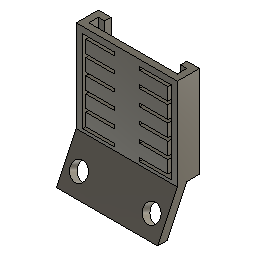
clip (Autodesk Fusion 360 design; units mm, degrees)
Autodesk Fusion 360 part; units mm, degrees
sketch "Skizze1" plane through (0, 0, 0) normal (1, 0, 0) x (0, 1, 0)
  line L0 (5, 36) -> (5, 7)
  line L1 (5, 7) -> (1, 7)
  line L2 (5, 36) -> (-2, 36)
  line L3 (-9.0346, 36) -> (15, -14) construction
  line L4 (-5.2641, -6.0314) -> (1, 7)
  line L5 (-2, 7) -> (-8.2641, -6.0314)
  line L6 (-8.2641, -6.0314) -> (-5.2641, -6.0314)
  line L7 (-2, 7) -> (-2, 36)
  constraint vertical L0
  constraint perpendicular L0 L1
  constraint horizontal L2
extrude "Extrusion2" add sketch "Skizze1" along normal mid plane 32 makes body 1
sketch "Skizze2" plane through (0, 0, 36) normal (0, 0, 1) x (-1, 0, 0)
  line L0 (-16, 2) -> (-16, -5)
  line L1 (-16, -5) -> (16, -5)
  line L2 (16, -5) -> (16, 2)
  line L3 (12, -3) -> (14, -3)
  line L4 (14, -3) -> (14, -1)
  line L5 (14, -1) -> (-14, -1)
  line L6 (-14, -1) -> (-14, -3)
  line L7 (-14, -3) -> (-12, -3)
  line L8 (-12, -3) -> (-12, -5)
  line L9 (12, -3) -> (12, -5)
  line L10 (12, -5) -> (-12, -5)
  line L11 (16, 2) -> (-16, 2)
  line L12 (12, -3) -> (-12, -3)
  constraint parallel L1 L3
  constraint perpendicular L1 L4
  constraint perpendicular L4 L5
  constraint perpendicular L1 L6
  constraint perpendicular L6 L7
  constraint coincident L1 L8.end
  constraint perpendicular L1 L8
  constraint coincident L1 L9.end
  constraint perpendicular L1 L9
  constraint perpendicular L8 L12
extrude "Extrusion3" cut sketch "Skizze2" against normal blind 28 contours L1 L8 L9 L10 L12 | L3 L4 L5 L6 L7 L12 bodies 1
sketch "Skizze3" plane through (0, -2, 0) normal (0, -1, 0) x (1, 0, 0)
  line L0 (-4, 29) -> (-4, 28)
  line L1 (-4, 28) -> (-13, 28)
  line L2 (-13, 28) -> (-13, 24)
  line L3 (-13, 24) -> (-4, 24)
  line L4 (-4, 24) -> (-4, 23)
  line L5 (-4, 23) -> (-13, 23)
  line L6 (-13, 23) -> (-13, 19)
  line L7 (-13, 19) -> (-4, 19)
  line L8 (-4, 19) -> (-4, 18)
  line L9 (-4, 18) -> (-13, 18)
  line L10 (-13, 18) -> (-13, 14)
  line L11 (-13, 14) -> (-4, 14)
  line L12 (-4, 14) -> (-4, 13)
  line L13 (-4, 13) -> (-13, 13)
  line L14 (-13, 13) -> (-13, 9)
  line L15 (-13, 9) -> (-4, 9)
  line L16 (-4, 9) -> (-4, 8)
  line L17 (-4, 8) -> (-14, 8)
  line L18 (-4, 29) -> (-13, 29)
  line L19 (-13, 29) -> (-13, 33)
  line L20 (-13, 33) -> (-4, 33)
  line L21 (-4, 33) -> (-4, 34)
  line L22 (-4, 34) -> (-14, 34)
  line L23 (-14, 34) -> (-14, 8)
  line L24 (4, 9) -> (4, 8)
  line L25 (4, 23) -> (13, 23)
  line L26 (4, 18) -> (13, 18)
  line L27 (4, 8) -> (14, 8)
  line L28 (13, 18) -> (13, 14)
  line L29 (4, 14) -> (4, 13)
  line L30 (14, 34) -> (14, 8)
  line L31 (13, 23) -> (13, 19)
  line L32 (4, 28) -> (13, 28)
  line L33 (4, 33) -> (4, 34)
  line L34 (13, 28) -> (13, 24)
  line L35 (13, 19) -> (4, 19)
  line L36 (13, 29) -> (13, 33)
  line L37 (13, 33) -> (4, 33)
  line L38 (4, 34) -> (14, 34)
  line L39 (4, 24) -> (4, 23)
  line L40 (4, 29) -> (4, 28)
  line L41 (13, 9) -> (4, 9)
  line L42 (4, 19) -> (4, 18)
  line L43 (13, 13) -> (13, 9)
  line L44 (4, 13) -> (13, 13)
  line L45 (13, 14) -> (4, 14)
  line L46 (13, 24) -> (4, 24)
  line L47 (4, 29) -> (13, 29)
  line L48 (-16, 7) -> (16, 7)
  line L49 (16, 7) -> (16, 36)
  line L50 (16, 36) -> (-16, 36)
  line L51 (-16, 36) -> (-16, 7)
  constraint perpendicular L0 L1
  constraint perpendicular L1 L2
  constraint perpendicular L0 L3
  constraint perpendicular L1 L4
  constraint perpendicular L0 L5
  constraint perpendicular L1 L6
  constraint perpendicular L6 L7
  constraint perpendicular L7 L8
  constraint perpendicular L6 L9
  constraint perpendicular L9 L10
  constraint perpendicular L6 L11
  constraint perpendicular L11 L12
  constraint perpendicular L12 L13
  constraint perpendicular L11 L14
  constraint perpendicular L14 L15
  constraint perpendicular L11 L16
  constraint perpendicular L16 L17
  constraint perpendicular L0 L18
  constraint perpendicular L18 L19
  constraint perpendicular L0 L20
  constraint perpendicular L20 L21
  constraint perpendicular L0 L22
  constraint perpendicular L17 L23
extrude "Extrusion4" cut sketch "Skizze3" against normal blind 3 contours L0 L1 L2 L3 L4 L5 L6 L7 L8 L9 L10 L11 L12 L13 L14 L15 L16 L17 L18 L19 L20 L21 L22 L23 | L24 L25 L26 L27 L28 L29 L30 L31 L32 L33 L34 L35 L36 L37 L38 L39 L40 L41 L42 L43 L44 L45 L46 L47 bodies 1
sketch "Skizze4" plane through (-13, 0, 0) normal (-1, 0, 0) x (0, -1, 0)
  spline S0 degree 5 poles (-0.6, 30) (-0.5838, 30.0067) (-0.5435, 30.0228) (-0.4594, 30.0556) (-0.3079, 30.1256) (-0.0957, 30.3027) (0.0811, 30.5925) (0.1688, 30.9921) (0.1107, 31.3665) (-0.0858, 31.6037) (-0.3409, 31.7375) (-0.5133, 31.8156) (-0.5842, 31.895) (-0.6, 31.9626) (-0.6, 32) knots 0 0 0 0 0 0 0.1 0.2 0.3 0.4 0.5 0.6 0.7 0.8 0.9 1 1 1 1 1 1
  line L0 (-0.6964, 29.9603) -> (-0.5036, 30.0397)
  line L1 (-0.6, 31.7862) -> (-0.6, 32.2138)
  line L2 (0, 33.0963) -> (-1, 33.0963)
  line L3 (-1, 33.0963) -> (-1, 28.9104)
  line L4 (-1, 28.9104) -> (0.0216, 28.9)
  spline S1 degree 5 poles (0, 33.0963) (-0.088, 33.0955) (-0.2452, 33.0815) (-0.4251, 33.0227) (-0.5685, 32.8792) (-0.6408, 32.6278) (-0.6461, 32.3913) (-0.6303, 32.2005) (-0.6115, 32.0678) (-0.6, 32) knots 0 0 0 0 0 0 0.2 0.4 0.6 0.8 1 1 1 1 1 1
  spline S2 degree 5 poles (-0.6, 30) (-0.6103, 29.9321) (-0.6269, 29.7991) (-0.6395, 29.6079) (-0.63, 29.3708) (-0.553, 29.1186) (-0.4065, 28.9746) (-0.2248, 28.9153) (-0.0667, 28.9009) (0.0216, 28.9) knots 0 0 0 0 0 0 0.2 0.4 0.6 0.8 1 1 1 1 1 1
  line L5 (-0.1725, 28.902) -> (0.2157, 28.898)
  line L6 (0.1918, 33.0979) -> (-0.1918, 33.0947)
  line L7 (2, 33) -> (-1, 33)
  line L8 (-1, 33) -> (-1, 29)
  line L9 (-1, 29) -> (2, 29)
  line L10 (0.1152, 30.5456) -> (0.15, 31.413)
  line L11 (2, 29) -> (2, 33)
  point P0 (0.1326, 30.9793)
  constraint midpoint L0 S0.start
  constraint midpoint L1 S0.end
  constraint horizontal L2
  constraint perpendicular L2 L3
  constraint midpoint L4.end L5
  constraint midpoint L2.start L6
  constraint midpoint P0 L10
  constraint parallel L1 L8
sketch "Skizze5" plane through (0, 0, 0) normal (1, 0, 0) x (0, 1, 0)
  spline S0 degree 5 poles (8.9, 31.5) (8.8955, 31.5452) (8.8759, 31.634) (8.8148, 31.7629) (8.68, 31.9266) (8.4785, 32.1214) (8.3101, 32.3108) (8.2322, 32.4994) (8.2744, 32.6906) (8.4162, 32.8861) (8.6086, 33.0862) (8.7563, 33.2498) (8.841, 33.3743) (8.8828, 33.458) (8.9, 33.5) knots 0 0 0 0 0 0 0.1 0.2 0.3 0.4 0.5 0.6 0.7 0.8 0.9 1 1 1 1 1 1
  line L0 (8.9281, 31.2175) -> (8.8719, 31.7825)
  line L1 (8.7875, 33.2251) -> (9.0125, 33.7749)
  line L2 (9, 34) -> (9, 31)
  line L3 (8.9, 33.5) -> (9, 34)
  line L4 (8.9, 31.5) -> (9, 31)
  line L5 (11, 36) -> (11, 29)
  line L6 (11, 29) -> (9, 29)
  line L7 (9, 29) -> (9, 31)
  line L8 (11, 36) -> (9, 36)
  line L9 (9, 36) -> (9, 34)
  point P0 (8.2618, 32.5)
  constraint vertical L5
  constraint perpendicular L5 L6
  constraint perpendicular L5 L8
extrude "Extrusion6" add sketch "Skizze5" along normal mid plane 27 separate body makes body 2
extrude "Extrusion7" cut sketch "Skizze5" along normal mid plane 14 contours S0 L1 L2 L4 | L1 L2 L3 bodies 2
sketch "Skizze7" plane through (0, -1.921, 0.9234) normal (0, 0.90128, -0.433238) x (-1, 0, 0)
  line L0 (16, 7) -> (-16, 7)
  line L1 (-16, 7) -> (-16, -5)
  line L2 (-16, -5) -> (16, -5)
  line L3 (16, -5) -> (16, 7)
  circle A0 centre (11.5, -3) radius 2.75
  circle A1 centre (-11.5, -3) radius 2.75
  line L4 (16, 6.7422) -> (-16, 6.7422)
  line L5 (-16, 6.7422) -> (-16, -7.7165)
  line L6 (-16, -7.7165) -> (16, -7.7165)
  line L7 (16, -7.7165) -> (16, 6.7422)
  dimension "d19" = 5.5
  dimension "d20" = 5.5
  measures "d19" diameter of A0
  measures "d20" diameter of A1
extrude "Extrusion9" cut sketch "Skizze7" against normal blind 3 contours L2 A0 | L2 A0 | L2 A1 | L2 A1 bodies 1
extrude "Extrusion10" add sketch "Skizze4" against normal blind 9 separate body contours S0 L0 L3 S1 S2 L7 L8 L9 makes body 3
copy_body "Körper kopieren/einfügen10" bodies 3 makes body 4
move_body "Verschieben11" bodies 4 to x (1, 0, 0) y (0, 1, 0) z (0, 0, 1) at (0, 0, -5)
copy_body "Körper kopieren/einfügen11" bodies 3 4 makes body 5 makes body 6
move_body "Verschieben12" bodies 5 6 to x (1, 0, 0) y (0, 1, 0) z (0, 0, 1) at (0, 0, -10)
copy_body "Körper kopieren/einfügen12" bodies 6 makes body 7
move_body "Verschieben13" bodies 7 to x (1, 0, 0) y (0, 1, 0) z (0, 0, 1) at (0, 0, -5)
copy_body "Körper kopieren/einfügen13" bodies 3 5 6 7 4 makes body 8 makes body 9 makes body 10 makes body 11 makes body 12
move_body "Verschieben14" bodies 8 9 10 11 12 to x (1, 0, 0) y (0, 1, 0) z (0, 0, 1) at (17, 0, 0)
combine "Kombinieren3" operation cut target body 1 tool bodies 3 9 5 6 8 7 10 12 11 4
sketch "Skizze8" plane through (0, 0, 36) normal (0, 0, 1) x (-1, 0, 0)
  line L0 (12, -3) -> (12, -5)
  line L1 (12, -5) -> (16, -5)
  line L2 (16, -5) -> (16, 2)
  line L3 (-16, 2) -> (-16, -5)
  line L4 (-16, -5) -> (-12, -5)
  line L5 (-12, -5) -> (-12, -3)
  line L6 (-12, -3) -> (-14, -3)
  line L7 (-14, -3) -> (-14, -1)
  line L8 (-14, -1) -> (14, -1)
  line L9 (14, -1) -> (14, -3)
  line L10 (14, -3) -> (12, -3)
  line L11 (14, -1) -> (-14, -1)
  line L12 (-14, -1) -> (-14, 0)
  line L13 (-14, 0) -> (14, 0)
  line L14 (14, 0) -> (14, -1)
  line L15 (16, 2) -> (-16, 2)
  dimension "d27" = 28
  constraint horizontal L11
  constraint vertical L12
  constraint horizontal L13
  constraint vertical L14
  constraint coincident L8.end L9.start
  measures "d27" distance of L8.end L7.end
extrude "Extrusion11" cut sketch "Skizze8" against normal blind 3 contours L8 L11 L12 L13 L14 bodies 1
sketch "Skizze9" plane through (0, 0, 36) normal (0, 0, 1) x (-1, 0, 0)
  line L0 (13.5, -9) -> (-13.5, -9)
  line L1 (-13.5, -9) -> (-13.5, -11)
  line L2 (-13.5, -11) -> (13.5, -11)
  line L3 (13.5, -11) -> (13.5, -9)
  line L4 (11.5, -14) -> (-11.4841, -14)
  line L5 (-11.4841, -14) -> (-11.4841, -11)
  line L6 (-11.4841, -11) -> (11.5, -11)
  line L7 (11.5, -11) -> (11.5, -14)
  constraint horizontal L4
  constraint vertical L5
  constraint horizontal L6
  constraint vertical L7
  constraint coincident L2 L5.end
extrude "Extrusion12" add sketch "Skizze9" along normal blind -17 and the other way blind -12 contours L2 L4 L5 L6 L7 bodies 2
sketch "Skizze10" plane through (0, 14, 0) normal (0, 1, 0) x (-1, 0, 0)
  line L0 (-11.4841, 48) -> (-11.4841, 19)
  line L1 (-11.4841, 19) -> (11.5, 19)
  line L2 (11.5, 19) -> (11.5, 48)
  line L3 (11.5, 48) -> (-11.4841, 48)
  circle A0 centre (-8, 43.5) radius 1.75
  circle A1 centre (8, 43.5) radius 1.75
  circle A2 centre (-8, 23.5) radius 1.75
  circle A3 centre (8, 23.5) radius 1.75
  dimension "d34" = 3.5
  dimension "d35" = 3.5
  dimension "d36" = 3.5
  dimension "d37" = 3.5
  measures "d34" diameter of A0
  measures "d35" diameter of A1
  measures "d36" diameter of A2
  measures "d37" diameter of A3
extrude "Extrusion13" cut sketch "Skizze10" against normal blind 3 contours A0 | A1 | A2 | A3 bodies 2
extrude "Extrusion14" cut sketch "Skizze2" against normal blind 29 contours L1 L8 L9 L10 L12 bodies 1
hidden bodies 2
